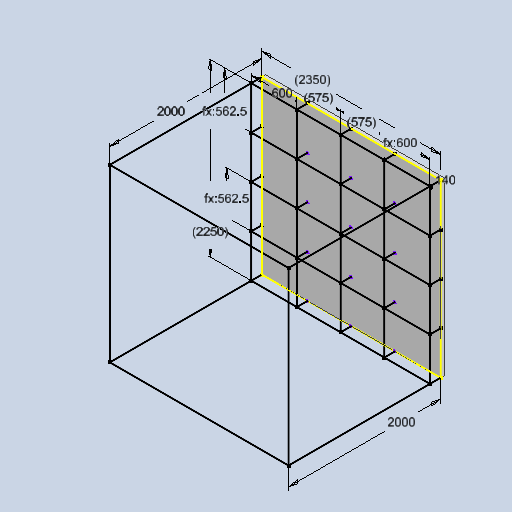
# Autodesk Inventor part: DF frame sketch v2.0
Saved by Autodesk Inventor 2025 (Build 290162010, 162A)
## iProperties
Created: 2023-08-31
Part Number: DF frame sketch v2.0
Material: Generic
Document SubType Name: Modeling
Designer: admin
Density: 1 g/cm^3
Appearance: Default
Author: admin
Autodesk Inventor part; units mm, degrees
ref_plane "YZ Plane" through (0, 0, 0) normal (1, 0, 0) x (0, 1, 0)
ref_plane "XZ Plane" through (0, 0, 0) normal (0, 1, 0) x (-1, 0, 0)
ref_plane "XY Plane" through (0, 0, 0) normal (0, 0, 1) x (1, 0, 0)
sketch "Sketch1" plane through (0, 0, 0) normal (0, 0, 1) x (1, 0, 0)
  line L0 (-1175, 1000) -> (1175, 1000)
  line L1 (1175, 1000) -> (1175, -1250)
  line L2 (1175, -1250) -> (-1175, -1250)
  line L3 (-1175, -1250) -> (-1175, 1000)
  line L4 (-1175, 1000) -> (1175, -1250) construction
  line L5 (1175, 1000) -> (-1175, -1250) construction
  point P0 (0, 0)
  point P1 (0, -125)
  dimension "d1" = 2350
  dimension "d5" = 1250
  dimension "d6" = 1000
  constraints: 12 end point, 2 midpoint, 2 parallel, 1 horizontal, 1 perpendicular, 1 vertical alignment
  measures "d1" distance of L0.start L0.end
  measures "d5" distance from line of L2 point (0, 0)
  measures "d6" distance from line of L0 point (0, 0)
extrude "Extrusion1" add sketch "Sketch1" against normal blind 50
sketch3d "3D Sketch1"
equation "\"d11\" = d10"
equation "\"d15\" = 0.25 * d18"
equation "\"d17\" = d15"
equation "\"d10\" = 600"
equation "\"d18\" = 2250"
body "Solid1"
